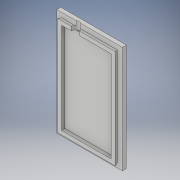
# Autodesk Inventor part: feeder_encolsure_lid
Saved by Autodesk Inventor 2019 (Build 230136000, 136)
## iProperties
Created: 2018-11-21
Part Number: feeder_encolsure_lid
Material: Generic
Document SubType Name: Modeling
Designer: chill
Density: 1 g/cm^3
Appearance: Default
Author: chill
Autodesk Inventor part; units mm, degrees
ref_plane "YZ Plane" through (0, 0, 0) normal (1, 0, 0) x (0, 1, 0)
ref_plane "XZ Plane" through (0, 0, 0) normal (0, 1, 0) x (-1, 0, 0)
ref_plane "XY Plane" through (0, 0, 0) normal (0, 0, 1) x (1, 0, 0)
sketch "Sketch1" plane through (0, 0, 0) normal (0, 0, 1) x (1, 0, 0)
  line L0 (0, 0) -> (36, 0)
  line L1 (36, 0) -> (36, -62)
  line L2 (36, -62) -> (0, -62)
  line L3 (0, -62) -> (0, 0)
  line L4 (-2.5, 2.5) -> (38.5, 2.5)
  line L5 (38.5, 2.5) -> (38.5, -64.5)
  line L6 (38.5, -64.5) -> (-2.5, -64.5)
  line L7 (-2.5, -64.5) -> (-2.5, 2.5)
  dimension "d0" = 36
  dimension "d1" = 62
  dimension "d2" = 2.5
  constraints: 16 end point, 4 parallel, 2 perpendicular, 1 horizontal, 3 other
  measures "d0" distance of L1.end L2.end
  measures "d1" distance of L0.end L1.end
  measures "d2" distance between parallel lines of L3 L7
extrude "Extrusion1" add sketch "Sketch1" along normal blind 2.5 contours L0 L1 L2 L3 | L4 L5 L6 L7
sketch "Sketch2" plane through (0, 0, 2.5) normal (0, 0, 1) x (1, 0, 0)
  line L0 (38.5, 2.5) -> (-2.5, 2.5) projected
  line L1 (-2.5, 2.5) -> (-2.5, -64.5) projected
  line L2 (-2.5, -64.5) -> (38.5, -64.5) projected
  line L3 (38.5, -64.5) -> (38.5, 2.5) projected
  line L4 (0, 0) -> (36, 0)
  line L5 (36, 0) -> (36, -62)
  line L6 (36, -62) -> (0, -62)
  line L7 (0, -62) -> (0, 0)
  line L8 (2.5, -2.5) -> (33.5, -2.5)
  line L9 (33.5, -2.5) -> (33.5, -59.5)
  line L10 (33.5, -59.5) -> (2.5, -59.5)
  line L11 (2.5, -59.5) -> (2.5, -2.5)
  point P0 (0, 0)
  dimension "d5" = 2.5
  dimension "d6" = 2.5
  constraints: 16 end point, 6 other
  measures "d5" distance between parallel lines of L0 L4
  measures "d6" distance between parallel lines of L7 L11
extrude "Extrusion2" add sketch "Sketch2" along normal blind 2 contours L4 L5 L6 L7
sketch "Sketch3" plane through (0, -62, 2.5) normal (-1, 0, 0) x (0, 0, 1)
  line L0 (0, 62) -> (2, 62) projected
  line L1 (0, 62) -> (0, 61.5)
  line L2 (0, 64.5) -> (0, -2.5) projected
  line L3 (2, 62) -> (2, 0) projected
  line L4 (0, 61.5) -> (2, 62)
  line L5 (2, 62) -> (0, 62)
  line L6 (0, 0) -> (0, 0.5)
  line L7 (0, 0) -> (0, 62) projected
  line L8 (0, 0.5) -> (2, 0)
  line L9 (0, 0) -> (2, 0) projected
  line L10 (2, 0) -> (0, 0)
  point P0 (-2.5, 62)
  dimension "d9" = 0.5
  dimension "d10" = 0.5
  constraints: 12 end point, 3 point on line, 1 collinear, 1 perpendicular
  measures "d9" distance of L0.start L1.end
  measures "d10" distance of L6.start L6.end
sketch "Sketch4" plane through (0, 0, 2.5) normal (0, 1, 0) x (1, 0, 0)
  line L0 (36, 0) -> (36, -2) projected
  line L1 (36, -2) -> (36, 0)
  line L2 (36, 0) -> (35.5, 0)
  line L3 (36, 0) -> (0, 0) projected
  line L4 (35.5, 0) -> (36, -2)
  line L5 (0, 0) -> (0, -2) projected
  line L6 (0, -2) -> (0, 0)
  line L7 (0, 0) -> (0.5, 0)
  line L8 (0.5, 0) -> (0, -2)
  point P0 (0, 2.5)
  dimension "d13" = 0.5
  dimension "d14" = 0.5
  constraints: 12 end point, 2 collinear, 2 point on line
  measures "d13" distance of L0.start L2.end
  measures "d14" distance of L3.end L7.end
extrude "Extrusion3" cut sketch "Sketch3" against normal through all contours L0 L4 L1 | L9 L2 L8
extrude "Extrusion4" cut sketch "Sketch4" against normal through all
sketch "Sketch5" plane through (-2.5, 2.5, 0) normal (0, 1, 0) x (1, 0, 0)
  line L0 (5, -4.5) -> (36, -4.5) projected
  line L1 (20.5, -4.5) -> (13.5, -4.5)
  circle A0 centre (13.5, -4.5) radius 2.5
  point P0 (2.5, 0)
  dimension "d17" = 7
  dimension "d18" = 5
  constraints: 2 end point, 1 centre point, 1 coincident, 1 midpoint, 1 point on line
  measures "d17" distance of L1.start L1.end
  measures "d18" diameter of A0
extrude "Extrusion5" cut sketch "Sketch5" against normal blind 5
fillet "Fillet1" radius 0.25 1 edges at (11, -2.5, 2.5)
body "Solid1"
